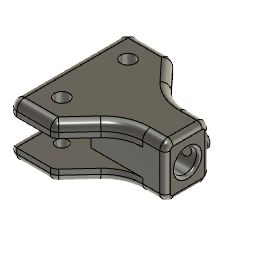
lampenhalter_v2 (Autodesk Fusion 360 design; units mm, degrees)
part number: 2026-05-11-20-10-54-553
Autodesk Fusion 360 part; units mm, degrees
note: some values were not read from the file. Chosen so that the rebuilt part matches the saved one: which bodies a step acts on; which face or edge a step refers to; which pieces of a blend or face edit are solid. Set by a fixed rule: which sketch regions a step uses.
sketch "Sketch1" plane through (0, 0, 0) normal (0, 0, 1) x (1, 0, 0)
  circle A0 centre (0, 0) radius 2.25
  circle A1 centre (0, 25) radius 2.25
  line L0 (-10, 35) -> (50, 35)
  line L1 (50, 35) -> (50, -10)
  line L2 (50, -10) -> (-10, -10)
  line L3 (-10, -10) -> (-10, 35)
  dimension "d1" = 4.5
  dimension "d2" = 4.5
  dimension "d3" = 25
  constraint coincident A0.centre origin
  constraint horizontal L0
  constraint vertical L1
  constraint horizontal L2
  constraint vertical L3
  measures "d1" diameter of A0
  measures "d2" diameter of A1
  measures "d3" distance of A0.centre A1.centre
extrude "Extrude1" add sketch "Sketch1" along normal blind 20 makes body 1
sketch "Sketch2" plane through (0, 0, 20) normal (0, 0, 1) x (-1, 0, 0)
  circle A0 centre (0, -25) radius 2.25
  circle A1 centre (0, 0) radius 2.25
  line L0 (10, 10) -> (-50, 10)
  line L1 (-50, 10) -> (-50, -35)
  line L2 (-50, -35) -> (10, -35)
  line L3 (10, -35) -> (10, 10)
  line L4 (-7, -35) -> (-7, 10) construction
  dimension "d6" = 7
  constraint coincident L2 L4.start
  constraint coincident L0 L4.end
  constraint perpendicular L0 L4
  measures "d6" distance of A0.centre L4
sketch "Sketch3" plane through (0, 35, 0) normal (0, 1, 0) x (-1, 0, 0)
  line L0 (-50, 0) -> (10, 0)
  line L1 (10, 0) -> (10, 20)
  line L2 (10, 20) -> (-50, 20)
  line L3 (-50, 20) -> (-50, 0)
  line L4 (-7, 20) -> (-7, 0)
  line L5 (10, 5) -> (-7, 5)
  line L6 (10, 15) -> (-7, 15)
  line L7 (-50, 20) -> (10, 20)
  point P0 (-7, 20)
  dimension "d7" = 5
  dimension "d8" = 5
  constraint coincident P0 L4.start
  constraint coincident L0 L4.end
  constraint perpendicular L0 L4
  constraint coincident L1 L5.start
  constraint coincident L4 L5.end
  constraint perpendicular L4 L5
  constraint coincident L1 L6.start
  constraint coincident L4 L6.end
  constraint perpendicular L4 L6
  measures "d7" distance of L0 L5
  measures "d8" distance of L6 L7
extrude "Extrude2" cut sketch "Sketch3" against normal blind 45 contours L1 L4 L5 L6 bodies 1
sketch "Sketch4" plane through (50, 0, 0) normal (1, 0, 0) x (0, 1, 0)
  line L0 (-10, 0) -> (35, 0)
  line L1 (35, 0) -> (35, 20)
  line L2 (35, 20) -> (-10, 20)
  line L3 (-10, 20) -> (-10, 0)
  line L4 (35, 10) -> (-10, 10) construction
  circle A0 centre (12.5, 10) radius 3.4
  circle A1 centre (12.5, 10) radius 4.35
  dimension "d11" = 6.8
  dimension "d12" = 8.7
  constraint midpoint L1 L4.start
  constraint midpoint L3 L4.end
  constraint midpoint L4 A0.centre
  constraint concentric A0 A1
  measures "d11" diameter of A0
  measures "d12" diameter of A1
extrude "Extrude3" cut sketch "Sketch4" against normal blind 10 contours A1 bodies 1
extrude "Extrude4" cut 1 faces at (50, 12.8369, 9.457) along direction (-1, 0, 0) blind 30 on bodies 1 bodies 1
sketch "Sketch5" plane through (40, 0, 0) normal (1, 0, 0) x (0, 1, 0)
  circle A0 centre (12.5, 10) radius 3.4
  circle A1 centre (12.5, 10) radius 4.35
  line L0 (9.5, 10.75) -> (8.1098, 10.75)
  line L1 (8.1098, 10.75) -> (8.1098, 9.25)
  line L2 (8.1098, 9.25) -> (9.5, 9.25)
  line L3 (9.5, 9.25) -> (9.5, 10.75)
  line L4 (12.5, 10) -> (7, 10) construction
  dimension "d17" = 1.5
  constraint horizontal L0
  constraint vertical L1
  constraint horizontal L2
  constraint vertical L3
  constraint coincident A0.centre A1.centre
  constraint perpendicular L3 L4
  constraint symmetric L0 L2 L4
  measures "d17" distance of L0 L2
extrude "Extrude5" cut sketch "Sketch5" against normal blind 30 contours A0 A1 L0 L2 picked at (8.8361, 9.4161) bodies 1
fillet "Fillet1" radius 1 1 edges at (50, 8.4444, 11.573) on bodies 1
fillet "Fillet2" radius 1 1 edges at (40, 15.9, 10) on bodies 1
sketch "Sketch6" plane through (50, 0, 0) normal (1, 0, 0) x (0, 1, 0)
  line L0 (-10, 0) -> (35, 0)
  line L1 (35, 0) -> (35, 20)
  line L2 (35, 20) -> (-10, 20)
  line L3 (-10, 20) -> (-10, 0)
  circle A0 centre (12.5, 10) radius 5.35
  line L4 (35, 0) -> (20, 0)
  line L5 (20, 0) -> (20, 20)
  line L6 (20, 20) -> (35, 20)
  line L7 (35, 20) -> (35, 0)
  line L8 (5, 0) -> (-10, 0)
  line L9 (-10, 0) -> (-10, 20)
  line L10 (-10, 20) -> (5, 20)
  line L11 (5, 20) -> (5, 0)
  constraint horizontal L4
  constraint vertical L5
  constraint horizontal L6
  constraint vertical L7
  constraint coincident L2 L5.end
  constraint coincident L0.end L1.start
  constraint horizontal L8
  constraint vertical L9
  constraint horizontal L10
  constraint vertical L11
  constraint coincident L2.end L3.start
  constraint coincident L0 L8.start
extrude "Extrude6" cut sketch "Sketch6" against normal blind 43 contours L0 L2 L3 L8 L9 L10 L11 | L0 L1 L2 L4 L5 L6 L7 bodies 1
extrude "Extrude7" add 1 faces at (35.6667, 20, 11.6667) along direction (0, 1, 0) blind 1 on bodies 1 bodies 1
extrude "Extrude8" add 1 faces at (35.6667, 5, 8.3333) along direction (0, -1, 0) blind 1 on bodies 1 bodies 1
sketch "Sketch7" plane through (0, 21, 0) normal (0, 1, 0) x (-1, 0, 0)
  line L0 (-50, 20) -> (-50, 0)
  line L1 (-50, 0) -> (-7, 0)
  line L2 (-7, 0) -> (-7, 5)
  line L3 (-7, 5) -> (-7, 15)
  line L4 (-7, 15) -> (-7, 20)
  line L5 (-7, 20) -> (-50, 20)
  circle A0 through (-42.8831, 10, -8.5) (-46.1081, 11.862, -8.5) (-46.1081, 8.138, -8.5)
  dimension "d32" = 4.3
sketch "Sketch7 (curves -8.5 mm off its plane)" plane through (0, 12.5, 0) normal (0, 1, 0) x (-1, 0, 0)
  circle A0 centre (-45.0331, 10) radius 2.15
extrude "Extrude9" cut sketch "Sketch7 (curves -8.5 mm off its plane)" along normal blind 9.5 bodies 1
sketch "Sketch8" plane through (0, 21, 0) normal (0, 1, 0) x (-1, 0, 0)
  circle A0 centre (-45.0331, 10) radius 2.15
  line L0 (-50, 20) -> (-50, 0)
  line L1 (-50, 0) -> (-7, 0)
  line L2 (-7, 0) -> (-7, 5)
  line L3 (-7, 5) -> (-7, 15)
  line L4 (-7, 15) -> (-7, 20)
  line L5 (-7, 20) -> (-50, 20)
  circle A1 centre (-45.0331, 10) radius 2.15
  circle A2 centre (-45.0331, 10) radius 3
  dimension "d35" = 6
  constraint concentric A0 A1
  constraint concentric A1 A2
  measures "d35" diameter of A2
extrude "Extrude10" add sketch "Sketch8" along normal blind 2 contours A2 bodies 1
sketch "Sketch9" plane through (0, 0, 20) normal (0, 0, 1) x (-1, 0, 0)
  circle A0 centre (0, 0) radius 2.25
  circle A1 centre (0, -25) radius 2.25
  line L0 (-7, 10) -> (-7, -4)
  line L1 (-50, -4) -> (-50, -21)
  line L2 (10, -35) -> (10, 10)
  circle A2 centre (0, 0) radius 2.75
  circle A3 centre (0, -25) radius 2.75
  line L3 (-7, -4) -> (-50, -4)
  line L4 (-50, -21) -> (-7, -21)
  line L5 (-7, -21) -> (-7, -35)
  line L6 (-7, -35) -> (10, -35)
  line L7 (10, 10) -> (-7, 10)
  dimension "d42" = 5.5
  dimension "d43" = 5.5
  constraint coincident A0.centre A2.centre
  constraint concentric A1 A3
  measures "d42" diameter of A2
  measures "d43" diameter of A3
extrude "Extrude11" cut sketch "Sketch9" against normal blind 4 contours A2 | A3 bodies 1
extrude "Extrude14" cut 1 faces at (20, 12.5264, 9.0645) along direction (-1, 0, 0) blind 19 on bodies 1 bodies 1
extrude "Extrude15" cut 1 faces at (10, 8.8361, 9.4161) along direction (-1, 0, 0) blind 16 on bodies 1 bodies 1
ref_plane "WorkPlane1" through (35, 0, 0) normal (1, 0, 0) x (0, 1, 0)
ref_plane "WorkPlane2" through (20, 0, 0) normal (1, 0, 0) x (0, 1, 0)
split "Split1" by plane through (35, 0, 0) normal (1, 0, 0) and through (20, 0, 0) normal (1, 0, 0) bodies 1 makes body 2 at (25, 21, 6.6667) makes body 3 at (45, 4, 13.3333)
delete_body "RemoveBody1" bodies 2
move_body "Move1" bodies 3 to x (1, 0, 0) y (0, 1, 0) z (0, 0, 1) at (-15, 0, 0)
combine "Combine1" operation add target body 1 tool bodies 3
sketch "Sketch11" plane through (0, 0, 0) normal (0, 0, -1) x (1, 0, 0)
  circle A0 centre (0, 0) radius 2.25
  circle A1 centre (0, -25) radius 2.25
  line L0 (35, -4) -> (7, -4)
  line L1 (7, -4) -> (7, 10)
  line L2 (7, 10) -> (-10, 10)
  line L3 (-10, 10) -> (-10, -35)
  line L4 (-10, -35) -> (7, -35)
  line L5 (7, -35) -> (7, -21)
  line L6 (7, -21) -> (35, -21)
  line L7 (35, -21) -> (35, -4)
  line L8 (10.3902, -12.5) -> (-10, -12.5) construction
  line L9 (7, -35) -> (20, -21)
  line L10 (7, 10) -> (20, -4)
  constraint midpoint L3 L8.end
  constraint perpendicular L3 L8
  constraint coincident L4.end L5.start
  constraint coincident L6 L9.end
  constraint symmetric L8 L4.end L1.end
  constraint symmetric L8 L9.end L10.end
extrude "Extrude16" add sketch "Sketch11" against normal blind 5 contours L0 L1 L10 | L5 L6 L9 bodies 1
sketch "Sketch12" plane through (0, 0, 20) normal (0, 0, 1) x (-1, 0, 0)
  line L0 (-35, -21) -> (-7, -21)
  line L1 (-7, -21) -> (-7, -35)
  line L2 (-7, -35) -> (10, -35)
  line L3 (10, -35) -> (10, 10)
  line L4 (10, 10) -> (-7, 10)
  line L5 (-7, 10) -> (-7, -4)
  line L6 (-7, -4) -> (-35, -4)
  line L7 (-35, -4) -> (-35, -21)
  circle A0 centre (0, 0) radius 2.75
  circle A1 centre (0, -25) radius 2.75
  line L8 (-7, -35) -> (-20, -21)
  line L9 (10, 10, -15) -> (10, -35, -15)
  line L10 (10, -35, -15) -> (10, -35, -20)
  line L11 (10, -35, -20) -> (10, 10, -20)
  line L12 (10, 10, -20) -> (10, 10, -15)
  line L13 (-10.3902, -12.5, -20) -> (10, -12.5, -17.5)
  line L14 (0, -12.5) -> (-10.5, -12.5) construction
  line L15 (-7, 10) -> (-20, -4)
  point P0 (-10.3902, -12.5)
  constraint horizontal L14
  constraint symmetric L1.end L14 L4.end
  constraint symmetric L8.end L14 L15.end
extrude "Extrude17" add sketch "Sketch12" against normal blind 5 contours L0 L1 L8 | L5 L6 L15 bodies 1
fillet "Fillet10" radius 15 4 edges at (20, 21, 2.5) (20, 21, 17.5) (20, 4, 2.5) (20, 4, 17.5) on bodies 1
fillet "Fillet11" radius 3 12 edges at (30.7705, 21, 0) (20.5453, 22.2504, 0) (11.2746, 30.3966, 0) (11.2746, 30.3966, 20) (20.5453, 22.2504, 20) (30.7705, 21, 20) (11.2746, -5.3966, 0) (20.5453, 2.7496, 0) (30.7705, 4, 0) (30.7705, 4, 20) (20.5453, 2.7496, 20) (11.2746, -5.3966, 20) on bodies 1
fillet "Fillet12" radius 3 12 edges at (7, 35, 16) (5.8009, 35, 19.1213) (-3.547, 35, 20) (-3.547, 35, 0) (5.8009, 35, 0.8787) (7, 35, 4) (-3.547, -10, 20) (5.8009, -10, 19.1213) (7, -10, 16) (7, -10, 4) (5.8009, -10, 0.8787) (-3.547, -10, 0) on bodies 1
fillet "Fillet13" radius 3 2 faces at (-10, 19, 16.6667) (-10, 19, 3.3333) on bodies 1
fillet "Fillet14" radius 2 8 edges at (35, 12.5, 0) (35, 4.8787, 0.8787) (35, 4, 10) (35, 4.8787, 19.1213) (35, 12.5, 20) (35, 20.1213, 19.1213) (35, 21, 10) (35, 20.1213, 0.8787) on bodies 1
fillet "Fillet15" radius 1 2 edges at (33.0331, 20.9997, 10) (27.0331, 21, 10) on bodies 1
